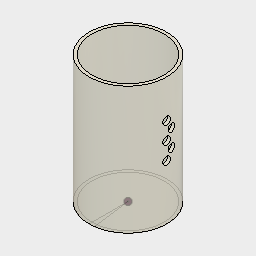
lfom (Autodesk Fusion 360 design; units mm, degrees)
Autodesk Fusion 360 part; units mm, degrees
sketch "Sketch1" plane through (0, 0, 0) normal (0, 1, 0) x (1, 0, 0)
  circle A0 centre (0, 0) radius 152.4
  circle A1 centre (0, 0) radius 140.6769
  line L0 (0, 0) -> (19.9426, -151.0895)
  line L1 (0, 0) -> (0, -152.4)
  dimension "d25" = 7.519
  measures "d25" angle of L0 L1
extrude "Extrude1" add sketch "Sketch1" along normal blind 500 contours A0 A1 L0 L1 | A0 A1 L0 L1
sketch "Sketch2" plane through (0, 0, 0) normal (1, 0, 0) x (0, 0, -1)
  circle A0 centre (0, 215) radius 15
  circle A1 centre (0, 257.5) radius 15
  circle A2 centre (0, 300) radius 15
  circle A3 centre (0, 342.5) radius 15
  circle A4 centre (0, 385) radius 15
extrude "lfom_hole_1" cut sketch "Sketch2" along normal through all contours A0
pattern_linear "seed_1" count 3 spacing 68 along (0, 1, 0) of 1 faces at (144.2655, 226.5282, -9.597)
ref_plane "WorkPlane1" through (0, 0, 0) normal (0.991401, 0, -0.130857) x (0, 1, 0)
sketch "Sketch3" plane through (0, 0, 0) normal (0.991401, 0, -0.130857) x (0, 1, 0)
  circle A0 centre (249, 0) radius 15
extrude "lfom_hole_2" cut sketch "Sketch3" along normal through all
pattern_linear "seed_2" count 2 spacing 68 along (0, 1, 0) of 1 faces at (143.1992, 234.0355, -19.942)
equation "od = 12\"" comment "Outer Diameter"
equation "sdr = 26" comment "Standard Dimensional Ratio (od/thickness_pipe)"
equation "oal = 0.5 m" comment "Over All Length"
equation "d4 = od"
equation "d5 = od / sdr"
equation "d6 = oal"
equation "h_holes = 20 cm"
equation "id_holes = 3 cm"
equation "n_rows = 5"
equation "b_bottom = 0.2 m" comment "The buffer between the bottom of the pipe and the beginning of the holes"
equation "d12 = id_holes"
equation "d13 = b_bottom + id_holes / 2"
equation "d18 = n_rows"
equation "d20 = h_holes - id_holes"
equation "d21 = ceil(n_rows / 2)"
equation "d23 = _d_v_center_holes * 2"
equation "d25 = _a_offset"
equation "d26 = id_holes"
equation "d27 = b_bottom + id_holes / 2 + _d_v_center_holes"
equation "d29 = floor(n_rows / 2)"
equation "d31 = _d_v_center_holes * 2"
equation "b_edge_holes = 1 cm" comment "The buffer between the edge of each hole. This is the width of the piece of pipe remaining"
equation "_a_offset = ( _d_h_center / ( od / 2 ) ) * 1 rad" comment "The angle off the center row the second row is."
equation "_d_h_center = ( id_holes + b_edge_holes ) / 2" comment "Horizontal distance center to center of holes"
equation "_d_v_center_holes = ( h_holes - id_holes ) / n_rows" comment "Real vertical center to center distance of hole rows"
equation "n_max_hole_per_row = floor(( od * 3.141 ) / ( id_holes + b_edge_holes ))" comment "This is the max number of holes we could put in the pipe while keeping the specified buffer"
